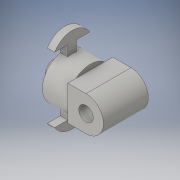
# Autodesk Inventor part: Germi01-03-01
Saved by Autodesk Inventor 2016 (Build 200138000, 138)
## iProperties
Created: 2016-11-08
Part Number: Germi01-03-01
Material: Generic
Document SubType Name: Modeling
Designer: Kai
Density: 1 g/cm^3
Appearance: Default
Author: Kai
Autodesk Inventor part; units mm, degrees
ref_plane "YZ Plane" through (0, 0, 0) normal (1, 0, 0) x (0, 1, 0)
ref_plane "XZ Plane" through (0, 0, 0) normal (0, 1, 0) x (-1, 0, 0)
ref_plane "XY Plane" through (0, 0, 0) normal (0, 0, 1) x (1, 0, 0)
sketch "Sketch1" plane through (0, 0, 0) normal (0, 1, 0) x (-1, 0, 0)
  line L0 (0, 15.4608) -> (12.8016, 15.4608)
  line L1 (12.8016, 15.4608) -> (12.8016, -0.338)
  line L2 (12.8016, -0.338) -> (0, -0.338)
  line L3 (0, -0.338) -> (0, 15.4608)
  constraints: 8 end point, 2 horizontal, 1 perpendicular, 1 vertical
extrude "Extrusion1" add sketch "Sketch1" along normal blind 12.192
sketch "Sketch2" plane through (-12.8016, 0, 15.4608) normal (0, 0, 1) x (1, 0, 0)
  arc A0 (6.4008, 0) -> (6.4008, 12.192) centre (6.4008, 6.096) ccw
  line L0 (0, 12.192) -> (12.8016, 12.192) projected
  line L1 (12.8016, 0) -> (0, 0) projected
  line L2 (6.4008, 0) -> (17.5033, -4.1356)
  line L3 (17.5033, -4.1356) -> (19.4121, 8.0167)
  line L4 (19.4121, 8.0167) -> (11.5072, 13.7088)
  line L5 (11.5072, 13.7088) -> (6.4008, 12.192)
  constraints: 8 end point, 2 midpoint, 2 point on circle, 1 centre point, 1 tangent
extrude "Extrusion2" cut sketch "Sketch2" along normal mid plane 2540
sketch "Sketch3" plane through (-12.8016, 0, 15.4608) normal (0, 0, 1) x (1, 0, 0)
  arc A0 (6.4008, 0) -> (6.4008, 12.192) centre (6.4008, 6.096) ccw projected
  circle A1 centre (6.4008, 6.096) radius 2.54
  point P0 (12.8016, 0)
  dimension "d8" = 5.08
  constraints: 1 centre point, 1 coincident
  measures "d8" diameter of A1
extrude "Extrusion3" cut sketch "Sketch3" against normal blind 2540
sketch "Sketch4" plane through (-12.8016, 0, -0.338) normal (-1, 0, 0) x (0, 0, 1)
  circle A0 centre (7.8994, 6.096) radius 7.8994
  point P0 (0.338, 0)
  constraints: 1 centre point
extrude "Extrusion4" add sketch "Sketch4" along normal blind 8.89
sketch "Sketch5" plane through (-21.6916, 6.096, 7.5614) normal (-1, 0, 0) x (0, 0, 1)
  circle A0 centre (0, 0) radius 7.8994 projected
  line L0 (-7.8994, 0) -> (7.8994, 0)
  line L1 (1.5587, -11.4554) -> (1.5587, -7.7441)
  line L2 (-1.5587, -7.7441) -> (-1.5587, -11.4554)
  line L3 (-6.1592, -11.4554) -> (-1.5587, -11.4554)
  line L4 (1.5587, -11.4554) -> (6.1592, -11.4554)
  arc A1 (-6.1592, -11.4554) -> (6.1592, -11.4554) centre (0, -7.8994) ccw
  line L5 (-1.5587, -7.7441) -> (1.5587, -7.7441)
  line L6 (1.5587, 7.7441) -> (-1.5587, 7.7441)
  line L7 (1.5587, 7.7441) -> (1.5587, 11.4554)
  line L8 (-1.5587, 11.4554) -> (-1.5587, 7.7441)
  line L9 (-1.5587, 11.4554) -> (-6.1592, 11.4554)
  arc A2 (6.1592, 11.4554) -> (-6.1592, 11.4554) centre (0, 7.8994) ccw
  line L10 (6.1592, 11.4554) -> (1.5587, 11.4554)
  point P0 (-7.5614, -6.096)
  dimension "d16" = 360
  constraints: 22 end point, 8 point on circle, 4 perpendicular, 2 centre point, 2 horizontal, 2 parallel, 27 other
extrude "Extrusion5" add sketch "Sketch5" against normal blind 2.54 contours L6 A0 | A0 L8 L9 A2 L10 L7 | L1 L4 A1 L3 L2 A0
sketch "Sketch6" plane through (-21.6916, 0, -0.338) normal (-1, 0, 0) x (0, 0, 1)
  arc A0 (2.8755, 12.192) -> (0, 6.096) centre (7.8994, 6.096) ccw projected
  circle A1 centre (7.8994, 6.096) radius 2.54
  point P0 (0.338, 0)
  dimension "d20" = 5.08
  constraints: 1 centre point, 1 coincident
  measures "d20" diameter of A1
extrude "Extrusion6" add sketch "Sketch6" along normal blind 2.54
sketch "Sketch7" plane through (-24.2316, 6.096, 7.5614) normal (-1, 0, 0) x (0, 0, 1)
  circle A0 centre (0, 0) radius 3.175
  point P0 (-7.5614, -6.096)
  dimension "d23" = 6.35
  constraints: 1 centre point
  measures "d23" diameter of A0
extrude "Extrusion7" add sketch "Sketch7" along normal blind 1.27
sketch "Sketch8" plane through (-25.5016, 6.096, 7.5614) normal (-1, 0, 0) x (0, 0, 1)
  point P0 (-7.5614, -6.096)
body "Solid1"
